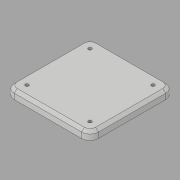
# Autodesk Inventor part: 2-2-5
Saved by Autodesk Inventor 2019 (Build 230136000, 136)
## iProperties
Created: 2020-11-06
Part Number: 2-2-5
Material: 一般
Document SubType Name: Modeling
Designer: Sugar
Density: 1 g/cm^3
Appearance: 預設
Author: Sugar
Autodesk Inventor part; units mm, degrees
ref_plane "YZ Plane" through (0, 0, 0) normal (1, 0, 0) x (0, 1, 0)
ref_plane "XZ Plane" through (0, 0, 0) normal (0, 1, 0) x (-1, 0, 0)
ref_plane "XY Plane" through (0, 0, 0) normal (0, 0, 1) x (1, 0, 0)
sketch "草圖1" plane through (0, 0, 0) normal (0, 1, 0) x (-1, 0, 0)
  line L0 (150, -150) -> (-150, -150)
  line L1 (-150, -150) -> (-150, 150)
  line L2 (-150, 150) -> (150, 150)
  line L3 (150, 150) -> (150, -150)
  point P0 (0, 0)
  point P1 (-150, 0)
  point P2 (0, -150)
  dimension "d0" = 300
  dimension "d1" = 300
  constraints: 8 end point, 2 midpoint, 2 parallel, 1 horizontal, 1 horizontal alignment, 1 perpendicular, 1 vertical alignment
  measures "d0" distance of L0.end L1.end
  measures "d1" distance of L1.end L2.end
extrude "擠出1" add sketch "草圖1" along normal mid plane 30
fillet "圓角1" radius 30 4 edges at (150, 0, 150) (150, 0, -150) (-150, 0, -150) (-150, 0, 150)
chamfer "倒角1" distance 10 angle 45 8 edges at (0, 15, 150) (141.2132, 15, 141.2132) (150, 15, 0) (141.2132, 15, -141.2132) (0, 15, -150) (-141.2132, 15, -141.2132) (-150, 15, 0) (-141.2132, 15, 141.2132)
sketch "草圖2" plane through (0, 15, 0) normal (0, 1, 0) x (1, 0, 0)
  line L0 (-112.5, 112.5) -> (112.5, 112.5) construction
  line L1 (112.5, 112.5) -> (112.5, -112.5) construction
  line L2 (112.5, -112.5) -> (-112.5, -112.5) construction
  line L3 (-112.5, -112.5) -> (-112.5, 112.5) construction
  point P0 (0, 0)
  point P1 (112.5, 0)
  point P2 (0, 112.5)
  dimension "d8" = 225
  dimension "d9" = 225
  constraints: 8 end point, 2 midpoint, 2 parallel, 1 horizontal, 1 horizontal alignment, 1 perpendicular, 1 vertical alignment
  measures "d8" distance of L0.start L0.end
  measures "d9" distance of L2.end L0.start
hole "孔1" at (-112.5, 15, -112.5) at (112.5, 15, -112.5) at (-112.5, 15, 112.5) at (112.5, 15, 112.5) direction (0, -1, 0) diameter 12 depth 10 tip angle 118
sketch "草圖3" plane through (0, -15, 0) normal (0, -1, 0) x (1, 0, 0)
  line L0 (125, 125) -> (-125, 125) construction
  line L1 (-125, 125) -> (-125, -125) construction
  line L2 (-125, -125) -> (125, -125) construction
  line L3 (125, -125) -> (125, 125) construction
  point P0 (0, 0)
  point P1 (0, -125)
  point P2 (125, 0)
  dimension "d19" = 250
  dimension "d20" = 250
  constraints: 8 end point, 2 midpoint, 2 parallel, 1 horizontal, 1 horizontal alignment, 1 perpendicular, 1 vertical alignment
  measures "d19" distance of L2.end L0.start
  measures "d20" distance of L1.end L2.end
hole "孔2" at (125, -15, 125) at (125, -15, -125) at (-125, -15, 125) at (-125, -15, -125) direction (0, 1, 0) diameter 12 depth 10 tip angle 118
